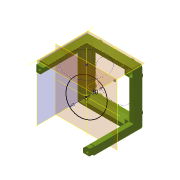
# Autodesk Inventor part: 10_Cube_1x1_IM
Saved by Autodesk Inventor 2019 (Build 230136000, 136)
## iProperties
Created: 2019-07-01
Part Number: 10_Cube_1x1_IM
Material: Generic
Document SubType Name: Modeling
Designer: diederichbenedict
Density: 1 g/cm^3
Appearance: IPHT_Grün
Mass: 11.4029 g
Surface Area: 91.4899 cm^2
Volume: 11.4029 cm^3
Author: diederichbenedict
Autodesk Inventor part; units mm, degrees
sketch "Sketch1" plane through (0, 0, 0) normal (0, 0, 1) x (1, 0, 0)
  line L0 (-24.85, 24.85) -> (24.85, 24.85)
  line L1 (24.85, 24.85) -> (24.85, -24.85)
  line L2 (24.85, -24.85) -> (-24.85, -24.85)
  line L3 (-24.85, -24.85) -> (-24.85, 24.85)
  line L4 (-24.85, 24.85) -> (24.85, -24.85) construction
  line L5 (24.85, 24.85) -> (-24.85, -24.85) construction
  line L6 (16.97, 16.97) -> (-16.97, 16.97)
  line L7 (-16.97, 16.97) -> (-16.97, -16.97)
  line L8 (-16.97, -16.97) -> (16.97, -16.97)
  line L9 (16.97, -16.97) -> (16.97, 16.97)
  point P0 (0, 0)
  dimension "d0" = 49.7
  dimension "d1" = 49.7
  dimension "d2" = 7.88
  constraints: 20 end point, 4 parallel, 2 midpoint, 2 perpendicular, 1 horizontal, 3 other
  measures "d0" distance of L1.end L2.end
  measures "d1" distance of L0.end L1.end
  measures "d2" distance between parallel lines of L0 L6
extrude "Extrusion1" add sketch "Sketch1" along normal blind 8
sketch "Sketch2" plane through (0, 0, 8) normal (0, 0, 1) x (1, 0, 0)
  line L0 (16.97, 16.97) -> (16.97, -16.97) projected
  line L1 (16.97, -16.97) -> (-16.97, -16.97) projected
  line L2 (-16.97, -16.97) -> (-16.97, 16.97) projected
  line L3 (-16.97, 16.97) -> (16.97, 16.97) projected
  line L4 (24.85, 24.85) -> (-24.85, 24.85) projected
  line L5 (-24.85, 24.85) -> (-24.85, -24.85) projected
  line L6 (-24.85, -24.85) -> (24.85, -24.85) projected
  line L7 (24.85, -24.85) -> (24.85, 24.85) projected
  line L8 (16.97, -16.97) -> (24.85, -16.97)
  line L9 (24.85, -16.97) -> (24.85, -24.85)
  line L10 (24.85, -24.85) -> (16.97, -24.85)
  line L11 (16.97, -24.85) -> (16.97, -16.97)
  line L12 (16.97, 16.97) -> (-16.97, 16.97) projected
  line L13 (24.85, 24.85) -> (16.97, 24.85)
  line L14 (16.97, 24.85) -> (16.97, 16.97)
  line L15 (16.97, 16.97) -> (24.85, 16.97)
  line L16 (24.85, 16.97) -> (24.85, 24.85)
  line L17 (-24.85, -24.85) -> (-16.97, -24.85)
  line L18 (-16.97, -24.85) -> (-16.97, -16.97)
  line L19 (-16.97, -16.97) -> (-24.85, -16.97)
  line L20 (-24.85, -16.97) -> (-24.85, -24.85)
  line L21 (-24.85, 24.85) -> (-16.97, 24.85)
  line L22 (-16.97, 24.85) -> (-16.97, 16.97)
  line L23 (-16.97, 16.97) -> (-24.85, 16.97)
  line L24 (-24.85, 16.97) -> (-24.85, 24.85)
  point P0 (0, 0)
  constraints: 32 end point, 8 parallel, 4 horizontal, 4 perpendicular
extrude "Extrusion2" add sketch "Sketch2" along normal blind 34.1 contours L14 L4 L7 L15 | L8 L7 L6 L11 | L23 L5 L4 L22 | L18 L6 L5 L19
sketch "Sketch3" plane through (0, 0, 0) normal (0, 0, -1) x (-1, 0, 0)
  line L0 (24.85, -24.85) -> (24.85, 24.85) construction
  line L1 (24.85, 24.85) -> (-24.85, 24.85) construction
  line L2 (-24.85, -24.85) -> (24.85, -24.85) construction
  line L3 (-24.85, 24.85) -> (-24.85, -24.85) construction
  point P0 (21.2, 21.2)
  point P1 (21.2, -21.2)
  point P2 (-21.2, -21.2)
  point P3 (-21.2, 21.2)
  dimension "d_1" = 3.65
  dimension "d96" = 3.65
  dimension "d97" = 3.65
  dimension "d98" = 3.65
  dimension "d99" = 3.65
  dimension "d100" = 3.65
  dimension "d101" = 3.65
  dimension "d102" = 3.65
  measures "d_1" distance from line of L1 point (21.2, 21.2)
  measures "d96" distance from line of point (21.2, 21.2) L0
  measures "d97" distance from line of point (21.2, -21.2) L0
  measures "d98" distance from line of point (21.2, -21.2) L2
  measures "d99" distance from line of point (-21.2, -21.2) L2
  measures "d100" distance from line of point (-21.2, -21.2) L3
  measures "d101" distance from line of point (-21.2, 21.2) L3
  measures "d102" distance from line of point (-21.2, 21.2) L1
hole "Hole1" at (-21.2, 21.2, 0) at (21.2, -21.2, 0) direction (0, 0, 1) diameter 3.1 depth 16 tip angle 118 counterbore diameter 5.5 counterbore depth 4.6
sketch "Sketch4" plane through (-24.85, 24.85, 0) normal (0, 1, 0) x (1, 0, 0)
  line L0 (0, 0) -> (49.7, 0) construction
  line L1 (0, 0) -> (0, -42.1) construction
  line L2 (7.88, -42.1) -> (0, -42.1) construction
  line L3 (7.88, -8) -> (7.88, -42.1) construction
  line L4 (41.82, -8) -> (7.88, -8) construction
  line L5 (41.82, -8) -> (41.82, -42.1) construction
  line L6 (49.7, -42.1) -> (41.82, -42.1) construction
  line L7 (49.7, 0) -> (49.7, -42.1) construction
  circle A0 centre (24.85, -24.97) radius 16.97 construction
  point P0 (24.85, 0)
  constraints: 3 tangent, 1 centre point
sketch "Sketch5" plane through (0, 0, 0) normal (0, 0, -1) x (-1, 0, 0)
  line L0 (-16.97, -16.97) -> (-16.97, 16.97) construction
  line L1 (-16.97, 16.97) -> (16.97, 16.97) construction
  line L2 (16.97, 16.97) -> (16.97, -16.97) construction
  line L3 (16.97, -16.97) -> (-16.97, -16.97) construction
  circle A0 centre (0, 0) radius 16.97 construction
  point P0 (0, 0)
  constraints: 3 tangent, 1 centre point
fillet "Fillet1" [suppressed]
sketch "Sketch6" plane through (0, 0, 42.1) normal (0, 0, 1) x (1, 0, 0)
  line L0 (-24.85, 24.85) -> (-24.85, 16.97) projected
  line L1 (-24.85, 16.97) -> (-16.97, 16.97) projected
  line L2 (-16.97, 16.97) -> (-16.97, 24.85) projected
  line L3 (-16.97, 24.85) -> (-24.85, 24.85) projected
  line L4 (24.85, 24.85) -> (16.97, 24.85) projected
  line L5 (16.97, 24.85) -> (16.97, 16.97) projected
  line L6 (16.97, 16.97) -> (24.85, 16.97) projected
  line L7 (24.85, 16.97) -> (24.85, 24.85) projected
  line L8 (24.85, -24.85) -> (24.85, -16.97) projected
  line L9 (24.85, -16.97) -> (16.97, -16.97) projected
  line L10 (16.97, -16.97) -> (16.97, -24.85) projected
  line L11 (16.97, -24.85) -> (24.85, -24.85) projected
  line L12 (-24.85, -24.85) -> (-16.97, -24.85) projected
  line L13 (-16.97, -24.85) -> (-16.97, -16.97) projected
  line L14 (-16.97, -16.97) -> (-24.85, -16.97) projected
  line L15 (-24.85, -16.97) -> (-24.85, -24.85) projected
  line L16 (0, 38.1838) -> (54, 38.1838) construction
  line L17 (20.75, 16.97) -> (16.97, 20.75)
  line L18 (16.97, 24.85) -> (16.97, 16.97) projected
  line L19 (16.97, 20.75) -> (16.97, 16.97)
  line L20 (16.97, 16.97) -> (20.75, 16.97)
  line L21 (-16.97, 24.85) -> (-16.97, 16.97) projected
  line L22 (-16.97, 16.97) -> (-16.97, 20.75)
  line L23 (-16.97, 20.75) -> (-20.75, 16.97)
  line L24 (-16.97, 20.75) -> (-11.6243, 20.75) construction
  line L25 (-16.97, -16.97) -> (-16.97, 16.97) projected
  line L26 (-20.75, 16.97) -> (-16.97, 16.97)
  line L27 (-16.97, 16.97) -> (-20.75, 16.97)
  line L28 (16.97, -16.97) -> (16.97, -24.85) projected
  line L29 (16.97, -16.97) -> (20.75, -16.97)
  line L30 (24.85, -16.97) -> (16.97, -16.97) projected
  line L31 (20.75, -16.97) -> (16.97, -20.75)
  line L32 (16.97, -16.97) -> (16.97, -20.75)
  line L33 (-16.97, -16.97) -> (-20.75, -16.97)
  line L34 (-16.97, -16.97) -> (-16.97, -24.85) projected
  line L35 (-16.97, -16.97) -> (-16.97, -20.75)
  line L36 (-20.75, -16.97) -> (-16.97, -20.75)
  dimension "d105" = 3.78
  dimension "d106" = 3.78
  dimension "d107" = 3.78
  dimension "d109" = 3.78
  dimension "d110" = 3.78
  dimension "d175" = 3.78
  dimension "d176" = 3.78
  constraints: 30 end point, 9 point on line, 3 collinear, 2 horizontal, 2 perpendicular, 1 equal length, 1 parallel, 1 vertical
  measures "d105" distance of L5.end L17.end
  measures "d106" distance of L5.end L17.start
  measures "d107" distance of L1.end L22.end
  measures "d109" distance of L35.end L13.end
  measures "d110" distance of L33.end L13.end
  measures "d175" distance of L9.end L31.end
  measures "d176" distance of L9.end L29.end
extrude "Extrusion3" cut sketch "Sketch6" against normal up to surface (34.1 mm away) contours L13 L36 L14 | L23 L2 L1 | L17 L6 L5 | L31 L10 L9
sketch "Sketch7" plane through (-24.85, 16.97, 8) normal (0, -1, 0) x (1, 0, 0)
  line L0 (41.82, 0) -> (49.82, 0) construction
  line L1 (41.82, -8) -> (41.82, 0) construction
  line L2 (7.88, -8) -> (7.88, 0) construction
  line L3 (-0.12, 0) -> (7.88, 0) construction
  line L4 (41.7793, 33.8563) -> (41.82, 0) construction
  line L5 (7.88, 0) -> (8.0247, 34.1328) construction
  line L6 (41.82, 0) -> (7.88, 0) construction
  circle A0 centre (24.8758, 16.9239) radius 16.9239 construction
  line L7 (24.8281, 54.9707) -> (-13.171, 16.8672) construction
  line L8 (24.9234, -21.123) -> (62.9226, 16.9805) construction
  line L9 (62.9226, 16.9805) -> (24.8281, 54.9707) construction
  line L10 (24.8281, 54.9707) -> (24.9234, -21.123) construction
  line L11 (-13.171, 16.8672) -> (62.9226, 16.9805) construction
  line L12 (24.8281, 54.9707) -> (78.6409, 54.9707) construction
  line L13 (46, 0) -> (41.82, 0)
  line L14 (46, 0) -> (41.82, -4.18)
  line L15 (41.82, 0) -> (41.7793, 33.8563)
  line L16 (41.82, 0) -> (41.82, -4.18)
  line L17 (46, 0) -> (41.82, 0)
  line L18 (41.82, 0) -> (46, 0)
  line L19 (7.88, 0) -> (3.7, 0)
  line L20 (3.7, 0) -> (7.88, -4.18)
  line L21 (7.88, -4.18) -> (7.88, 0)
  point P0 (44.386, 0)
  point P1 (43.5978, 0)
  dimension "d39" = 53.8
  dimension "d177" = 4.18
  dimension "d178" = 4.18
  dimension "d179" = 4.18
  dimension "d180" = 4.18
  constraints: 38 end point, 3 collinear, 3 point on line, 3 tangent, 2 midpoint, 1 centre point, 1 equal length, 1 horizontal, 1 parallel, 1 vertical
  measures "d39" distance of L8.start L7.end
  measures "d177" distance of L0.start L13.start
  measures "d178" distance of L0.start L14.end
  measures "d179" distance of L2.end L19.end
  measures "d180" distance of L20.end L2.end
extrude "Extrusion4" cut sketch "Sketch7" along normal up to surface (33.94 mm away)
sketch "Sketch8" plane through (16.97, -24.85, 8) normal (-1, 0, 0) x (0, 0, 1)
  line L0 (-4.18, 41.82) -> (0, 41.82) construction
  line L1 (-4.18, 7.88) -> (0, 7.88) construction
  line L2 (0, 7.88) -> (0, 3.7) construction
  line L3 (-4.18, 7.88) -> (0, 3.7)
  line L4 (0, 3.7) -> (0, 7.88)
  line L5 (0, 7.88) -> (-4.18, 7.88)
  line L6 (-4.18, 41.82) -> (0, 46)
  line L7 (-4.18, 41.82) -> (1.7314, 41.82) construction
  line L8 (0, 7.88) -> (0, 41.82)
  line L9 (0, 46) -> (0, 41.82)
  line L10 (0, 41.82) -> (-4.18, 41.82)
  line L11 (-5.9742, 2.0864) -> (-5.9742, 47.2133)
  line L12 (-8, 49.7) -> (-8, 0) construction
  line L13 (-8, 49.7) -> (34.1, 49.7) construction
  line L14 (34.1, 41.82) -> (34.1, 49.7) construction
  line L15 (0, 41.82) -> (34.1, 41.82) construction
  line L16 (0, 7.88) -> (0, 41.82) construction
  line L17 (0, 7.88) -> (34.1, 7.88) construction
  line L18 (34.1, 0) -> (34.1, 7.88) construction
  line L19 (-8, 0) -> (34.1, 0) construction
  line L20 (0, 4.1) -> (0, 7.88) construction
  line L21 (0, 4.1) -> (0, 0) construction
  line L22 (0, 0) -> (0, 4.1) construction
  line L23 (0, 7.88) -> (0, 4.1) construction
  line L24 (0, 49.7) -> (0, 45.6) construction
  point P0 (-2.4607, 7.9982)
  point P1 (-0.0623, 5.4502)
  dimension "d112" = 45
  dimension "d181" = 4.18
  dimension "d182" = 4.18
  dimension "d183" = 4.18
  constraints: 20 end point, 3 horizontal, 3 vertical, 2 collinear, 1 equal length, 1 perpendicular, 6 other
  measures "d112" angle of L7 L6
  measures "d181" distance of L3.start L4.end
  measures "d182" distance of L3.end L4.end
  measures "d183" distance of L0.end L0.start
ref_plane "Work Plane1" through (-20.32, -18.034, 19.8181) normal (-1, 0, 0) x (0, 0, 1)
extrude "Extrusion5" cut sketch "Sketch8" along normal up to surface (33.94 mm away)
sketch "Sketch9" plane through (0, 0, 42.1) normal (0, 0, 1) x (1, 0, 0)
  circle A0 centre (20.95, 20.95) radius 1.55 projected
  circle A1 centre (21.2, -21.2) radius 1.55 projected
  circle A2 centre (-20.95, -20.95) radius 1.55 projected
  circle A3 centre (-21.2, 21.2) radius 1.55 projected
  point P0 (18.6978, 19.486)
  point P1 (19.486, 18.6978)
  point P2 (19.486, -18.6978)
  point P3 (18.6978, -19.486)
  point P4 (-18.6978, -19.486)
  point P5 (-19.486, -18.6978)
  point P6 (-19.486, 18.6978)
  point P7 (-18.6978, 19.486)
  constraints: 4 other
hole "Hole2" at (20.95, 20.95, 42.1) at (-21.2, 21.2, 42.1) at (21.2, -21.2, 42.1) at (-20.95, -20.95, 42.1) direction (0, 0, -1) diameter 2.8 depth 12 tip angle 118
sketch "Sketch16" plane through (0, 0, 42.1) normal (0, 0, 1) x (1, 0, 0)
  circle A0 centre (-20.95, -20.95) radius 1.4 projected
  line L0 (-16.97, -20.75) -> (-20.75, -16.97) projected
  line L1 (-20.75, -16.97) -> (-24.85, -16.97) projected
  line L2 (-24.85, -16.97) -> (-24.85, -24.85) projected
  line L3 (-24.85, -24.85) -> (-16.97, -24.85) projected
  line L4 (-16.97, -24.85) -> (-16.97, -20.75) projected
  circle A1 centre (20.95, 20.95) radius 1.4 projected
  line L5 (16.97, 20.75) -> (20.75, 16.97) projected
  line L6 (20.75, 16.97) -> (24.85, 16.97) projected
  line L7 (24.85, 16.97) -> (24.85, 24.85) projected
  line L8 (24.85, 24.85) -> (16.97, 24.85) projected
  line L9 (16.97, 24.85) -> (16.97, 20.75) projected
  point P0 (0, 0)
extrude "Extrusion6" cut sketch "Sketch16" against normal up to surface (34.1 mm away) contours A0 | L4 L3 L2 L1 L0 | A1 | L9 L8 L7 L6 L5
sketch "Sketch17" plane through (0, 0, 42.1) normal (0, 0, 1) x (1, 0, 0)
  circle A0 centre (-21.2, 21.2) radius 2.75 construction
  circle A1 centre (-21.2, 21.2) radius 1.4 projected
  line L0 (-20.75, 16.97) -> (-16.97, 20.75) construction
  line L1 (-16.97, 20.75) -> (-16.97, 24.85) construction
  line L2 (-16.97, 24.85) -> (-24.85, 24.85) construction
  line L3 (-24.85, 24.85) -> (-24.85, 16.97) construction
  line L4 (-24.85, 16.97) -> (-20.75, 16.97) construction
  circle A2 centre (21.2, -21.2) radius 1.4 construction
  line L5 (20.75, -16.97) -> (16.97, -20.75) construction
  line L6 (16.97, -20.75) -> (16.97, -24.85) construction
  line L7 (16.97, -24.85) -> (24.85, -24.85) construction
  line L8 (24.85, -24.85) -> (24.85, -16.97) construction
  line L9 (24.85, -16.97) -> (20.75, -16.97) construction
  line L10 (-20.07, 17.65) -> (-23.75, 17.65)
  line L11 (-23.75, 17.65) -> (-23.75, 23.75)
  line L12 (-23.75, 23.75) -> (-17.65, 23.75)
  line L13 (-17.65, 23.75) -> (-17.65, 20.07)
  line L14 (-20.75, 16.97) -> (-16.97, 20.75) projected
  line L15 (-20.07, 17.65) -> (-17.65, 20.07)
  line L16 (-20.95, -20.95) -> (20.95, 20.95) construction
  circle A3 centre (21.2, -21.2) radius 2.75 construction
  circle A4 centre (21.2, -21.2) radius 1.4
  line L17 (16.97, -20.75) -> (20.75, -16.97) construction
  line L18 (20.75, -16.97) -> (24.85, -16.97) construction
  line L19 (24.85, -16.97) -> (24.85, -24.85) construction
  line L20 (24.85, -24.85) -> (16.97, -24.85) construction
  line L21 (16.97, -24.85) -> (16.97, -20.75) construction
  line L22 (17.65, -20.07) -> (17.65, -23.75)
  line L23 (17.65, -23.75) -> (23.75, -23.75)
  line L24 (23.75, -23.75) -> (23.75, -17.65)
  line L25 (23.75, -17.65) -> (20.07, -17.65)
  line L26 (16.97, -20.75) -> (20.75, -16.97)
  line L27 (17.65, -20.07) -> (20.07, -17.65)
  point P0 (0, 0)
  dimension "d171" = 6.1
  dimension "d172" = 6.1
  dimension "d173" = 1.1
  dimension "d174" = 1.1
  constraints: 34 end point, 7 symmetric about line, 4 point on line, 3 perpendicular, 2 centre point, 1 collinear, 1 horizontal, 2 other
  measures "d171" distance between parallel lines of L12 L10
  measures "d172" distance between parallel lines of L13 L11
  measures "d173" distance between parallel lines of L3 L11
  measures "d174" distance between parallel lines of L2 L12
extrude "Extrusion7" add sketch "Sketch17" along normal blind 3.7
sketch "Sketch18" plane through (0, 0, 8) normal (0, 0, 1) x (1, 0, 0)
  line L0 (20.6727, 17.65) -> (23.75, 17.65)
  line L1 (23.75, 17.65) -> (23.75, 23.75)
  line L2 (23.75, 23.75) -> (17.65, 23.75)
  line L3 (17.65, 23.75) -> (17.65, 20.9704)
  line L4 (17.65, 20.9704) -> (20.6727, 17.65)
  circle A0 centre (21.2, 21.2) radius 1.55
  line L5 (-17.65, -20.6727) -> (-17.65, -23.75)
  line L6 (-17.65, -23.75) -> (-23.75, -23.75)
  line L7 (-23.75, -23.75) -> (-23.75, -17.65)
  line L8 (-23.75, -17.65) -> (-20.9704, -17.65)
  line L9 (-20.9704, -17.65) -> (-17.65, -20.6727)
  circle A1 centre (-21.2, -21.2) radius 1.55
  dimension "d164" = 3.1
  dimension "d169" = 6.1
  dimension "d170" = 6.1
  constraints: 20 end point, 2 centre point
  measures "d164" diameter of A0
  measures "d169" distance between parallel lines of L3 L1
  measures "d170" distance between parallel lines of L2 L0
extrude "Extrusion8" cut sketch "Sketch18" against normal blind 4.2 contours L4 L3 L2 L1 L0 | A0 | L5 L6 L7 L8 L9 | A1
fillet "Fillet2" radius 2 4 edges at (24.85, -24.85, 21.05) (24.85, 24.85, 4) (-24.85, 24.85, 21.05) (-24.85, -24.85, 4)
fillet "Fillet2" radius 0.5 24 edges at (23.75, -17.65, 43.95) (23.75, -23.75, 43.95) (20.07, -17.65, 43.95) (-17.65, 23.75, 43.95) (-17.65, 20.07, 43.95) (-23.75, 23.75, 43.95) (-23.75, 17.65, 43.95) (-20.07, 17.65, 43.95) (17.65, -20.07, 43.95) (17.65, -23.75, 43.95) (23.75, 23.75, 5.9) (20.6727, 17.65, 5.9) (17.65, 20.9704, 5.9) (17.65, 23.75, 5.9) (23.75, 17.65, 5.9) (0, 24.85, 0) (24.85, 0, 0) (-24.85, 0, 0) (0, -24.85, 0) (-20.9704, -17.65, 5.9) (-23.75, -17.65, 5.9) (-17.65, -20.6727, 5.9) (-17.65, -23.75, 5.9) (-23.75, -23.75, 5.9)
sketch "Sketch19" plane through (0, 0, 0) normal (0, 0, -1) x (-1, 0, 0)
  line L0 (16.97, 21.15) -> (-16.97, 21.15) construction
  line L1 (-16.97, -16.97) -> (-16.97, 16.97) construction
  line L2 (-16.97, 16.97) -> (16.97, 16.97) construction
  line L3 (16.97, 16.97) -> (16.97, -16.97) construction
  line L4 (16.97, -16.97) -> (-16.97, -16.97) construction
  circle A0 centre (21.2, 21.2) radius 2.75 construction
  circle A1 centre (-21.2, -21.2) radius 2.75 construction
  arc A2 (-24.35, -22.85) -> (-22.85, -24.35) centre (-22.85, -22.85) ccw construction
  line L5 (22.85, -24.35) -> (-22.85, -24.35) construction
  arc A3 (22.85, -24.35) -> (24.35, -22.85) centre (22.85, -22.85) ccw construction
  line L6 (24.35, 22.85) -> (24.35, -22.85) construction
  arc A4 (24.35, 22.85) -> (22.85, 24.35) centre (22.85, 22.85) ccw construction
  line L7 (-22.85, 24.35) -> (22.85, 24.35) construction
  arc A5 (-22.85, 24.35) -> (-24.35, 22.85) centre (-22.85, 22.85) ccw construction
  line L8 (-24.35, -22.85) -> (-24.35, 22.85) construction
  line L9 (-11.5874, 0) -> (13.4878, 0) construction
  line L10 (0, 12.1668) -> (0, -14.2062) construction
  line L11 (8.8, 20.66) -> (-8.8, 20.66) construction
  line L12 (8.8, 22.36) -> (-8.8, 22.36)
  line L13 (-8.8, 18.96) -> (8.8, 18.96)
  arc A6 (8.8, 18.96) -> (8.8, 22.36) centre (8.8, 20.66) ccw
  arc A7 (-8.8, 22.36) -> (-8.8, 18.96) centre (-8.8, 20.66) ccw
  line L14 (-18.96, -8.8) -> (-18.96, 8.8)
  line L15 (-20.66, 8.8) -> (-20.66, -8.8) construction
  line L16 (-22.36, 8.8) -> (-22.36, -8.8)
  arc A8 (-18.96, 8.8) -> (-22.36, 8.8) centre (-20.66, 8.8) ccw
  arc A9 (-22.36, -8.8) -> (-18.96, -8.8) centre (-20.66, -8.8) ccw
  line L17 (8.8, -18.96) -> (-8.8, -18.96)
  line L18 (-8.8, -20.66) -> (8.8, -20.66) construction
  line L19 (-8.8, -22.36) -> (8.8, -22.36)
  arc A10 (-8.8, -18.96) -> (-8.8, -22.36) centre (-8.8, -20.66) ccw
  arc A11 (8.8, -22.36) -> (8.8, -18.96) centre (8.8, -20.66) ccw
  line L20 (18.96, 8.8) -> (18.96, -8.8)
  line L21 (20.66, -8.8) -> (20.66, 8.8) construction
  line L22 (22.36, -8.8) -> (22.36, 8.8)
  arc A12 (18.96, -8.8) -> (22.36, -8.8) centre (20.66, -8.8) ccw
  arc A13 (22.36, 8.8) -> (18.96, 8.8) centre (20.66, 8.8) ccw
  point P0 (0, 0)
  point P1 (0, 0)
  point P2 (0, 20.66)
  point P3 (-20.66, 0)
  point P4 (0, -20.66)
  point P5 (20.66, 0)
  dimension "d134" = 3.4
  dimension "d135" = 21
  dimension "d136" = 7.38
  dimension "d137" = 3.69
  dimension "d140" = 360
  constraints: 36 end point, 16 point on circle, 8 centre point, 4 tangent, 3 point on line, 1 horizontal, 1 midpoint, 1 parallel, 1 perpendicular, 1 vertical, 49 other
  measures "d134" distance between parallel lines of L13 L12
  measures "d136" distance between parallel lines of L2 L7
  measures "d137" distance from line of L7 point (0, 20.66)
extrude "Extrusion9" cut sketch "Sketch19" against normal blind 4
sketch "Sketch20" plane through (0, 0, 0) normal (0, 0, -1) x (-1, 0, 0)
  arc A0 (-8.8, -18.96) -> (-8.8, -22.36) centre (-8.8, -20.66) ccw construction
  line L0 (-8.8, -18.96) -> (8.8, -18.96) construction
  arc A1 (8.8, -22.36) -> (8.8, -18.96) centre (8.8, -20.66) ccw construction
  line L1 (8.8, -22.36) -> (-8.8, -22.36) construction
  arc A2 (-8.8, 22.36) -> (-8.8, 18.96) centre (-8.8, 20.66) ccw construction
  line L2 (-8.8, 22.36) -> (8.8, 22.36) construction
  arc A3 (8.8, 18.96) -> (8.8, 22.36) centre (8.8, 20.66) ccw construction
  line L3 (8.8, 18.96) -> (-8.8, 18.96) construction
  arc A4 (-18.96, 8.8) -> (-22.36, 8.8) centre (-20.66, 8.8) ccw construction
  line L4 (-18.96, 8.8) -> (-18.96, -8.8) construction
  arc A5 (-22.36, -8.8) -> (-18.96, -8.8) centre (-20.66, -8.8) ccw construction
  line L5 (-22.36, -8.8) -> (-22.36, 8.8) construction
  arc A6 (18.96, -8.8) -> (22.36, -8.8) centre (20.66, -8.8) ccw construction
  line L6 (18.96, -8.8) -> (18.96, 8.8) construction
  arc A7 (22.36, 8.8) -> (18.96, 8.8) centre (20.66, 8.8) ccw construction
  line L7 (22.36, 8.8) -> (22.36, -8.8) construction
  line L8 (-16.97, -16.97) -> (-16.97, 16.97) construction
  line L9 (-16.97, 16.97) -> (16.97, 16.97) construction
  line L10 (16.97, 16.97) -> (16.97, -16.97) construction
  line L11 (16.97, -16.97) -> (-16.97, -16.97) construction
  circle A8 centre (21.2, 21.2) radius 2.75 construction
  circle A9 centre (-21.2, -21.2) radius 2.75 construction
  arc A10 (-24.35, -22.85) -> (-22.85, -24.35) centre (-22.85, -22.85) ccw construction
  line L12 (22.85, -24.35) -> (-22.85, -24.35) construction
  arc A11 (22.85, -24.35) -> (24.35, -22.85) centre (22.85, -22.85) ccw construction
  line L13 (24.35, 22.85) -> (24.35, -22.85) construction
  arc A12 (24.35, 22.85) -> (22.85, 24.35) centre (22.85, 22.85) ccw construction
  line L14 (-22.85, 24.35) -> (22.85, 24.35) construction
  arc A13 (-22.85, 24.35) -> (-24.35, 22.85) centre (-22.85, 22.85) ccw construction
  line L15 (-24.35, -22.85) -> (-24.35, 22.85) construction
  circle A14 centre (-14.3, 20.66) radius 2.475
  circle A15 centre (-14.3, 20.66) radius 1.025
  line L16 (8.8, 20.66) -> (-17.1249, 20.66) construction
  line L17 (0, -34.79) -> (0, 34.79) construction
  circle A16 centre (14.3, 20.66) radius 2.475
  circle A17 centre (14.3, 20.66) radius 1.025
  circle A18 centre (-20.66, -14.3) radius 1.025
  circle A19 centre (-20.66, -14.3) radius 2.475
  circle A20 centre (-20.66, 14.3) radius 1.025
  circle A21 centre (-20.66, 14.3) radius 2.475
  circle A22 centre (14.3, -20.66) radius 1.025
  circle A23 centre (14.3, -20.66) radius 2.475
  circle A24 centre (-14.3, -20.66) radius 1.025
  circle A25 centre (-14.3, -20.66) radius 2.475
  circle A26 centre (20.66, 14.3) radius 1.025
  circle A27 centre (20.66, 14.3) radius 2.475
  circle A28 centre (20.66, -14.3) radius 1.025
  circle A29 centre (20.66, -14.3) radius 2.475
  point P0 (0, 0)
  point P1 (17.1249, 20.66)
  point P2 (-20.66, -17.1249)
  point P3 (-20.66, 17.1249)
  point P4 (17.1249, -20.66)
  point P5 (-17.1249, -20.66)
  point P6 (20.66, 17.1249)
  point P7 (20.66, -17.1249)
  dimension "d144" = 4.95
  dimension "d145" = 2.05
  dimension "d146" = 5.5
  dimension "d149" = 360
  constraints: 16 centre point, 8 coincident, 3 symmetric about line, 2 end point, 2 point on line, 1 horizontal, 43 other
  measures "d144" diameter of A14
  measures "d145" diameter of A15
  measures "d146" distance of A2.centre A14.centre
extrude "Extrusion10" add sketch "Sketch20" along normal blind 2.2
ref_plane "Work Plane2" through (0, -16.97, 42.1) normal (1, 0, 0) x (0, 0, -1)
ref_plane "Work Plane3" through (-16.97, 0, 42.1) normal (0, 1, 0) x (1, 0, 0)
sketch "Sketch21" plane through (0, 0, 0) normal (0, 0, -1) x (-1, 0, 0)
  circle A0 centre (20.66, 14.3) radius 2.475 construction
  circle A1 centre (14.3, -20.66) radius 2.475 construction
  circle A2 centre (-20.66, -14.3) radius 2.475 construction
  circle A3 centre (-14.3, 20.66) radius 2.475 construction
  circle A4 centre (14.3, 20.66) radius 2.475 construction
  circle A5 centre (-20.66, 14.3) radius 2.475 construction
  circle A6 centre (-14.3, -20.66) radius 2.475 construction
  circle A7 centre (20.66, -14.3) radius 2.475 construction
  arc A8 (-8.8, -18.96) -> (-8.8, -22.36) centre (-8.8, -20.66) ccw construction
  line L0 (-8.8, -18.96) -> (8.8, -18.96) construction
  arc A9 (8.8, -22.36) -> (8.8, -18.96) centre (8.8, -20.66) ccw construction
  line L1 (8.8, -22.36) -> (-8.8, -22.36) construction
  arc A10 (-8.8, 22.36) -> (-8.8, 18.96) centre (-8.8, 20.66) ccw construction
  line L2 (-8.8, 22.36) -> (8.8, 22.36) construction
  arc A11 (8.8, 18.96) -> (8.8, 22.36) centre (8.8, 20.66) ccw construction
  line L3 (8.8, 18.96) -> (-8.8, 18.96) construction
  arc A12 (-18.96, 8.8) -> (-22.36, 8.8) centre (-20.66, 8.8) ccw construction
  line L4 (-18.96, 8.8) -> (-18.96, -8.8) construction
  arc A13 (-22.36, -8.8) -> (-18.96, -8.8) centre (-20.66, -8.8) ccw construction
  line L5 (-22.36, -8.8) -> (-22.36, 8.8) construction
  arc A14 (18.96, -8.8) -> (22.36, -8.8) centre (20.66, -8.8) ccw construction
  line L6 (18.96, -8.8) -> (18.96, 8.8) construction
  arc A15 (22.36, 8.8) -> (18.96, 8.8) centre (20.66, 8.8) ccw construction
  line L7 (22.36, 8.8) -> (22.36, -8.8) construction
  line L8 (-16.97, -16.97) -> (-16.97, 16.97) construction
  line L9 (-16.97, 16.97) -> (16.97, 16.97) construction
  line L10 (16.97, 16.97) -> (16.97, -16.97) construction
  line L11 (16.97, -16.97) -> (-16.97, -16.97) construction
  circle A16 centre (-21.2, -21.2) radius 2.75 construction
  circle A17 centre (21.2, 21.2) radius 2.75 construction
  arc A18 (-24.35, -22.85) -> (-22.85, -24.35) centre (-22.85, -22.85) ccw construction
  line L12 (22.85, -24.35) -> (-22.85, -24.35) construction
  arc A19 (22.85, -24.35) -> (24.35, -22.85) centre (22.85, -22.85) ccw construction
  line L13 (24.35, 22.85) -> (24.35, -22.85) construction
  arc A20 (24.35, 22.85) -> (22.85, 24.35) centre (22.85, 22.85) ccw construction
  line L14 (-22.85, 24.35) -> (22.85, 24.35) construction
  arc A21 (-22.85, 24.35) -> (-24.35, 22.85) centre (-22.85, 22.85) ccw construction
  line L15 (-24.35, -22.85) -> (-24.35, 22.85) construction
  circle A22 centre (-21.2, -21.2) radius 1.55 construction
  line L16 (21.2, 21.2) -> (-21.2, 21.2) construction
  line L17 (-21.2, 21.2) -> (-21.2, -21.2) construction
  line L18 (-21.2, -21.2) -> (21.2, -21.2) construction
  line L19 (21.2, -21.2) -> (21.2, 21.2) construction
  point P0 (0, 0)
  constraints: 8 end point, 2 parallel, 1 horizontal, 1 perpendicular
hole "Hole9" at (-21.2, -21.2, 0) at (21.2, 21.2, 0) direction (0, 0, 1) diameter 3.1 depth 16 tip angle 118 counterbore diameter 5.5 counterbore depth 3.2
sketch "Sketch22" plane through (0, 0, 0) normal (0, 0, -1) x (-1, 0, 0)
  circle A0 centre (21.2, -21.2) radius 2.75 construction
  circle A1 centre (-21.2, 21.2) radius 2.75 construction
  circle A2 centre (20.66, 14.3) radius 2.475 construction
  circle A3 centre (14.3, -20.66) radius 2.475 construction
  circle A4 centre (-20.66, -14.3) radius 2.475 construction
  circle A5 centre (-14.3, 20.66) radius 2.475 construction
  circle A6 centre (14.3, 20.66) radius 2.475 construction
  circle A7 centre (-20.66, 14.3) radius 2.475 construction
  circle A8 centre (-14.3, -20.66) radius 2.475 construction
  circle A9 centre (20.66, -14.3) radius 2.475 construction
  arc A10 (-8.8, -18.96) -> (-8.8, -22.36) centre (-8.8, -20.66) ccw construction
  line L0 (-8.8, -18.96) -> (8.8, -18.96) construction
  arc A11 (8.8, -22.36) -> (8.8, -18.96) centre (8.8, -20.66) ccw construction
  line L1 (8.8, -22.36) -> (-8.8, -22.36) construction
  arc A12 (-8.8, 22.36) -> (-8.8, 18.96) centre (-8.8, 20.66) ccw construction
  line L2 (-8.8, 22.36) -> (8.8, 22.36) construction
  arc A13 (8.8, 18.96) -> (8.8, 22.36) centre (8.8, 20.66) ccw construction
  line L3 (8.8, 18.96) -> (-8.8, 18.96) construction
  arc A14 (-18.96, 8.8) -> (-22.36, 8.8) centre (-20.66, 8.8) ccw construction
  line L4 (-18.96, 8.8) -> (-18.96, -8.8) construction
  arc A15 (-22.36, -8.8) -> (-18.96, -8.8) centre (-20.66, -8.8) ccw construction
  line L5 (-22.36, -8.8) -> (-22.36, 8.8) construction
  arc A16 (18.96, -8.8) -> (22.36, -8.8) centre (20.66, -8.8) ccw construction
  line L6 (18.96, -8.8) -> (18.96, 8.8) construction
  arc A17 (22.36, 8.8) -> (18.96, 8.8) centre (20.66, 8.8) ccw construction
  line L7 (22.36, 8.8) -> (22.36, -8.8) construction
  line L8 (-16.97, -16.97) -> (-16.97, 16.97) construction
  line L9 (-16.97, 16.97) -> (16.97, 16.97) construction
  line L10 (16.97, 16.97) -> (16.97, -16.97) construction
  line L11 (16.97, -16.97) -> (-16.97, -16.97) construction
  circle A18 centre (-21.2, -21.2) radius 2.75 construction
  circle A19 centre (21.2, 21.2) radius 2.75 construction
  arc A20 (-24.35, -22.85) -> (-22.85, -24.35) centre (-22.85, -22.85) ccw construction
  line L12 (22.85, -24.35) -> (-22.85, -24.35) construction
  arc A21 (22.85, -24.35) -> (24.35, -22.85) centre (22.85, -22.85) ccw construction
  line L13 (24.35, 22.85) -> (24.35, -22.85) construction
  arc A22 (24.35, 22.85) -> (22.85, 24.35) centre (22.85, 22.85) ccw construction
  line L14 (-22.85, 24.35) -> (22.85, 24.35) construction
  arc A23 (-22.85, 24.35) -> (-24.35, 22.85) centre (-22.85, 22.85) ccw construction
  line L15 (-24.35, -22.85) -> (-24.35, 22.85) construction
  line L16 (22.0219, -24.2672) -> (18.9546, -23.4454)
  line L17 (18.9546, -23.4454) -> (18.1328, -20.3781)
  line L18 (18.1328, -20.3781) -> (20.3781, -18.1328)
  line L19 (20.3781, -18.1328) -> (23.4454, -18.9546)
  line L20 (23.4454, -18.9546) -> (24.2672, -22.0219)
  line L21 (24.2672, -22.0219) -> (22.0219, -24.2672)
  line L22 (21.2, 21.2) -> (-21.2, -21.2) construction
  circle A24 centre (21.2, -21.2) radius 1.55 construction
  line L23 (-21.2, 21.2) -> (21.2, -21.2) construction
  line L24 (-24.2672, 22.0219) -> (-23.4454, 18.9546)
  line L25 (-23.4454, 18.9546) -> (-20.3781, 18.1328)
  line L26 (-20.3781, 18.1328) -> (-18.1328, 20.3781)
  line L27 (-18.1328, 20.3781) -> (-18.9546, 23.4454)
  line L28 (-18.9546, 23.4454) -> (-22.0219, 24.2672)
  line L29 (-22.0219, 24.2672) -> (-24.2672, 22.0219)
  point P0 (0, 0)
  dimension "d160" = 5.5
  dimension "d161" = 90
  constraints: 28 end point, 6 symmetric about line, 1 coincident, 1 perpendicular, 13 other
  measures "d160" distance between parallel lines of L18 L21
  measures "d161" angle of L23 L18
extrude "Extrusion11" cut sketch "Sketch22" against normal up to surface (3.2 mm away)
ref_plane "Work Plane4" through (-24.85, 24.85, 8) normal (-0.7071, -0.7071, 0) x (0, 0, 1)
sketch "Sketch23" plane through (-24.85, 24.85, 8) normal (-0.7071, -0.7071, 0) x (0, 0, 1)
  circle A0 centre (17.053, -35.1432) radius 15
  point P0 (-8, -35.1432)
  dimension "d184" = 30
  constraints: 1 centre point
  measures "d184" diameter of A0
ref_plane "Work Plane5" through (-16.97, 25.05, 42.1) normal (0, 1, 0) x (1, 0, 0)
ref_plane "Work Plane6" through (-25.05, 16.97, 8) normal (-1, 0, 0) x (0, 0, 1)
ref_plane "Arbeitsebene7" through (0, 0, 25.05) normal (0, 0, 1) x (1, 0, 0)
equation "\"d96\" = d_1"
equation "\"d97\" = d_1"
equation "\"d98\" = d_1"
equation "\"d99\" = d_1"
equation "\"d100\" = d_1"
equation "\"d101\" = d_1"
equation "\"d102\" = d_1"
body "Solid1"
